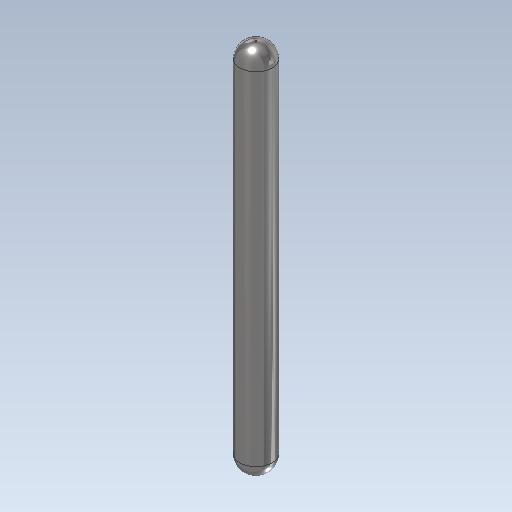
# Autodesk Inventor part: 1-47a000_023x263F
Saved by Autodesk Inventor 2020 (Build 240168000, 168)
## iProperties
Created: 2011-06-21
Part Number: 1-47a000_023x263F
Document SubType Name: Modeling
Designer: MarkN
Mass: 0.0139381 g
Surface Area: 0.122868 cm^2
Volume: 0.00174226 cm^3
Density: 8 g/cm^3
Material: Stainless Steel
Appearance: Semi-Polished
Author: MarkN
Autodesk Inventor part; units mm, degrees
ref_plane "YZ Plane" through (0, 0, 0) normal (1, 0, 0) x (0, 1, 0)
ref_plane "XZ Plane" through (0, 0, 0) normal (0, 1, 0) x (-1, 0, 0)
ref_plane "XY Plane" through (0, 0, 0) normal (0, 0, 1) x (1, 0, 0)
sketch "Sketch1-<F>" plane through (0, 0, 0) normal (0, 0, 1) x (1, 0, 0)
  circle A0 centre (0, 0) radius 0.2921
  dimension "d3" = 0.5842
  constraints: 1 centre point, 1 other
  measures "d3" diameter of A0
extrude "ExtrusionMidplane1" add sketch "Sketch1-<F>" along normal mid plane 6.6802
fillet "Fillet1" radius 0.2794 2 edges at (-0.2921, 0, -3.3401) (-0.2921, 0, 3.3401)
equation "\"mdt_d0\" = 0"
body "Solid1"
